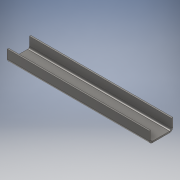
# Autodesk Inventor part: Cprofiel
Saved by Autodesk Inventor 2017 (Build 210142000, 142)
## iProperties
RuleStatus: InUse
Created: 2017-01-05
Part Number: Cprofiel
Material: Steel, Mild
Document SubType Name: Sheet Metal
Designer: bramp
Density: 7.85 g/cm^3
Flat Pattern Width: 8.87991 cm
Flat Pattern Length: 30 cm
Flat Pattern Area: 266.397 cm^2
Sheet Metal Rule: Default
Sheet Metal Width: 88,799 mm
Sheet Metal Length: 300,000 mm
Sheet Metal Area: 26639,734 mm^2
Appearance: Semi-Polished
Author: bramp
Autodesk Inventor part; units mm, degrees
ref_plane "YZ Plane" through (0, 0, 0) normal (1, 0, 0) x (0, 1, 0)
ref_plane "XZ Plane" through (0, 0, 0) normal (0, 1, 0) x (-1, 0, 0)
ref_plane "XY Plane" through (0, 0, 0) normal (0, 0, 1) x (1, 0, 0)
sketch "Sketch1" plane through (0, 0, 0) normal (0, 0, 1) x (1, 0, 0)
  line L0 (0, 0) -> (-300, 0)
  line L1 (-300, 0) -> (-300, 50)
  line L2 (-300, 50) -> (0, 50)
  line L3 (0, 50) -> (0, 0)
  dimension "d0" = 50
  dimension "d1" = 300
  measures "d0" distance between parallel lines of L2 L0
  measures "d1" distance between parallel lines of L3 L1
extrude "Plate1" add sketch "Sketch1" along normal blind 3
sketch "Sketch2" plane through (-300, 47, 0) normal (0, 1, 0) x (-1, 0, 0)
  line L0 (-300, 0) -> (0, 0)
  line L1 (0, 0) -> (0, 25)
  line L2 (0, 25) -> (-300, 25)
  line L3 (-300, 25) -> (-300, 0)
  constraints: 6 end point, 1 horizontal, 1 perpendicular, 1 vertical
edge flange "Flange1" height 25 angle 90 thickness 3 bend radius 3.9 thickness toward (0, 1, 0) relief straight relief width 3 relief depth 1.5 corner gap 3.9 corner form 0 edges at (-150, 50, 3) (-150, 0, 3) wall of the first edge with corners at (0, 47, 0) (-300, 47, 0) (-300, 47, 25) (0, 47, 25)
bend "Bend1"
corner "Corner1"
equation "\"d3\" = BendReliefWidth"
equation "\"d4\" = BendReliefDepth"
equation "\"d5\" = MinimumRemnant"
equation "\"d6\" = BendRadius"
equation "\"d9\" = BendRadius"
equation "\"d10\" = CornerReliefSize"
equation "\"d11\" = GapSize"
equation "\"d12\" = JacobiRadiusSize"
equation "\"BendReliefWidth\" = Thickness"
equation "\"BendReliefDepth\" = 0.5 * Thickness"
equation "\"CornerReliefSize\" = 4 * Thickness"
equation "\"MinimumRemnant\" = 2 * Thickness"
equation "\"TransitionRadius\" = BendRadius"
equation "\"JacobiRadiusSize\" = BendRadius"
equation "\"GapSize\" = Thickness"
equation "\"d2\" = BendRadius"
equation "\"BendRadius\" = 3.9"
equation "\"Thickness\" = 3"
body "Solid1"
